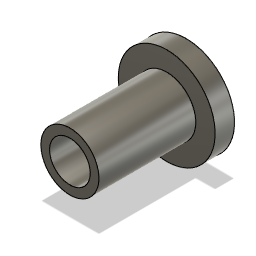
PTFE_Tube_Cap (Autodesk Fusion 360 design; units mm, degrees)
Autodesk Fusion 360 part; units mm, degrees
sketch "Skizze1" plane through (0, 0, 0) normal (0, 1, 0) x (1, 0, 0)
  circle A0 centre (0, 0) radius 5
  dimension "d1" = 10
  constraint coincident A0.centre origin
  measures "d1" diameter of A0
extrude "Extrusion1" add sketch "Skizze1" along normal blind 2
ref_plane "Arbeitsebene1" through (0, 2, 0) normal (0, 1, 0) x (-1, 0, 0)
sketch "Skizze3" plane through (0, 2, 0) normal (0, 1, 0) x (1, 0, 0)
  circle A0 centre (0, 0) radius 2.1
  circle A1 centre (0, 0) radius 3
  dimension "d7" = 4.2
  dimension "d8" = 6
  constraint coincident A0.centre A1.centre
  constraint concentric A0 A1
  measures "d7" diameter of A0
  measures "d8" diameter of A1
extrude "Extrusion2" add sketch "Skizze3" along normal blind 10
move_body "Verschieben1" bodies 1 to x (1, 0, 0) y (0, 0, 1) z (0, -1, 0) at (0, 2, -2)
